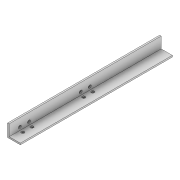
# Autodesk Inventor part: caleta_completa
Saved by Autodesk Inventor 2022 (Build 260153000, 153)
## iProperties
Created: 2022-11-13
Part Number: caleta_completa
Material: Genérico
Document SubType Name: Modeling
Designer: Jorge
Density: 1 g/cm^3
Appearance: Valor por defecto
Author: Jorge
Autodesk Inventor part; units mm, degrees
ref_plane "YZ Plane" through (0, 0, 0) normal (1, 0, 0) x (0, 1, 0)
ref_plane "XZ Plane" through (0, 0, 0) normal (0, 1, 0) x (-1, 0, 0)
sketch "Boceto1" plane through (0, 0, 0) normal (0, 0, 1) x (1, 0, 0)
  line L0 (0, 0) -> (0, 25)
  line L1 (0, 0) -> (25, 0)
  line L2 (3, 25) -> (3, 3)
  line L3 (3, 3) -> (25, 3)
  line L4 (0, 25) -> (3, 25)
  line L5 (25, 3) -> (25, 0)
  dimension "d0" = 25
  dimension "d1" = 25
  dimension "d2" = 3
  constraints: 12 end point, 2 horizontal, 2 vertical, 1 other
  measures "d0" distance of L0.start L0.end
  measures "d1" distance of L0.start L1.end
  measures "d2" distance between parallel lines of L0 L2
extrude "Extrusión1" add sketch "Boceto1" along normal blind 300
sketch "Boceto2" plane through (0, 0, 0) normal (0, -1, 0) x (1, 0, 0)
  line L0 (0, 0) -> (25, 0) construction
  line L1 (25, 0) -> (25, 300) construction
  line L2 (0, 300) -> (25, 300) construction
  line L3 (0, 0) -> (0, 300) construction
  line L4 (25, 0) -> (25, 300) construction
  line L5 (25, 150) -> (0, 150) construction
  line L6 (25, 300) -> (3, 300) projected
  line L7 (9, 300) -> (9, 0) construction
  circle A0 centre (9, 159) radius 1.6
  circle A1 centre (9, 141) radius 1.6
  circle A2 centre (9, 279) radius 1.6
  circle A3 centre (9, 261) radius 1.6
  line L8 (25, 270) -> (0, 270) construction
  line L9 (0, 0) -> (0, 300) construction
  dimension "d5" = 3.2
  dimension "d6" = 3.2
  dimension "d7" = 18
  dimension "d8" = 9
  dimension "d9" = 3.2
  dimension "d10" = 3.2
  dimension "d11" = 18
  dimension "d12" = 9
  dimension "d13" = 30
  dimension "d14" = 9
  constraints: 8 point on line, 6 end point, 4 centre point, 2 midpoint, 1 horizontal, 1 perpendicular
  measures "d5" diameter of A0
  measures "d6" diameter of A1
  measures "d7" distance of A1.centre A0.centre
  measures "d8" distance from line of L5 A0.centre
  measures "d9" diameter of A2
  measures "d10" diameter of A3
  measures "d11" distance of A3.centre A2.centre
  measures "d12" distance from line of L8 A2.centre
  measures "d13" distance between parallel lines of L2 L8
  measures "d14" distance between parallel lines of L3 L7
extrude "Extrusión2" cut sketch "Boceto2" against normal through all
ref_plane "Plano de trabajo1" through (0, 0, 0) normal (0.7071, -0.7071, 0) x (0, 0, 1)
mirror "Simetría1" about plane through (0, 0, 0) normal (0.7071, -0.7071, 0) of "Extrusión2"
sketch "Boceto3" plane through (3, 3, 0) normal (0, 1, 0) x (1, 0, 0)
  circle A0 centre (6, -279) radius 1.6 construction
  circle A1 centre (6, -141) radius 1.6 construction
  circle A2 centre (6, -159) radius 1.6 construction
  circle A3 centre (6, -261) radius 1.6 construction
  line L0 (22, 0) -> (0, 0) construction
  line L1 (0, 0) -> (0, -300) construction
  line L2 (22, -300) -> (0, -300) construction
  line L3 (22, 0) -> (22, -300) construction
  circle A4 centre (6, -141) radius 1.6 projected
  circle A5 centre (6, -141) radius 3
  circle A6 centre (6, -159) radius 1.6 projected
  circle A7 centre (6, -159) radius 3
  circle A8 centre (6, -261) radius 1.6 projected
  circle A9 centre (6, -261) radius 3
  circle A10 centre (6, -279) radius 1.6 projected
  circle A11 centre (6, -279) radius 3
  point P0 (-3, 0)
  dimension "d17" = 6
  dimension "d18" = 6
  dimension "d19" = 6
  dimension "d20" = 6
  constraints: 4 centre point, 4 coincident
  measures "d17" diameter of A5
  measures "d18" diameter of A7
  measures "d19" diameter of A9
  measures "d20" diameter of A11
extrude "Extrusión3" cut sketch "Boceto3" against normal blind 2 contours A4 | A5 | A6 | A7 | A8 | A9 | A10 | A11
mirror "Simetría2" about plane through (0, 0, 0) normal (0.7071, -0.7071, 0) of "Extrusión3"
equation "\"d8\" = 0.5 * d7"
equation "\"d12\" = 0.5 * d11"
